3.2mm thick (Autodesk Fusion 360 design; units mm, degrees)
Autodesk Fusion 360 part; units mm, degrees
note: some values were not read from the file. Chosen so that the rebuilt part matches the saved one: which bodies a step acts on. Set by a fixed rule: which sketch regions a step uses.
sketch "Sketch1" plane through (0, 0, 0) normal (0, 0, 1) x (1, 0, 0)
  line L0 (-28.9023, 0) -> (0, 0) construction
  line L1 (0, 0) -> (0, 16.228) construction
  line L2 (0, 16.228) -> (-28.9023, 16.228) construction
  line L3 (-28.9023, 16.228) -> (-28.9023, 0) construction
  dimension "d1" = 3
  text T0 "3.2 mm thick" font "Arial" height 3 align right bottom in box 28.9023 x 16.228 at (-28.9023, 0) x (1, 0) y (0, 1) spacing 1
  constraint coincident L0.end
extrude "Extrude1" add sketch "Sketch1" along normal blind 1 text T0 makes body 1 at (-16.3486, 1.1003, 0) makes body 2 at (-21.0266, 0.1398, 0.3333) makes body 3 at (-22.3325, 1.6191, 0) makes body 4 at (-1.8008, 1, 0.3333) makes body 5 at (-7.1603, 1, 0.3333) makes body 6 at (-4.8274, 0.7244, 0.3333) makes body 7 at (-3.7192, 0.4291, 0) makes body 8 at (-4.8274, 2.7176, 0.3333) makes body 9 at (-8.013, 1.0464, 0) makes body 10 at (-12.8574, 1.1003, 0) makes body 11 at (-19.2844, 0.118, 0)
sketch "Sketch2" plane through (0, 0, 0) normal (0, 0, 1) x (1, 0, 0)
  line L0 (-24, 3.9332) -> (0.4575, 3.9332)
  line L1 (0.4575, 3.9332) -> (0.4575, -1.8)
  line L2 (0.4575, -1.8) -> (-24, -1.8)
  line L3 (-24, -1.8) -> (-24, 3.9332)
  circle A0 centre (0.4575, 1.0666) radius 2.8666
  circle A1 centre (-24, 1.0666) radius 2.8666
  constraint horizontal L0
  constraint vertical L1
  constraint horizontal L2
  constraint vertical L3
  constraint coincident L1.end A0
  constraint tangent L2 A0
  constraint coincident L0.end A0
  constraint coincident L2.end A1
  constraint tangent L2 A1
  constraint coincident L0.start A1
extrude "Extrude2" add sketch "Sketch2" against normal blind 1 bodies 1 2 3
